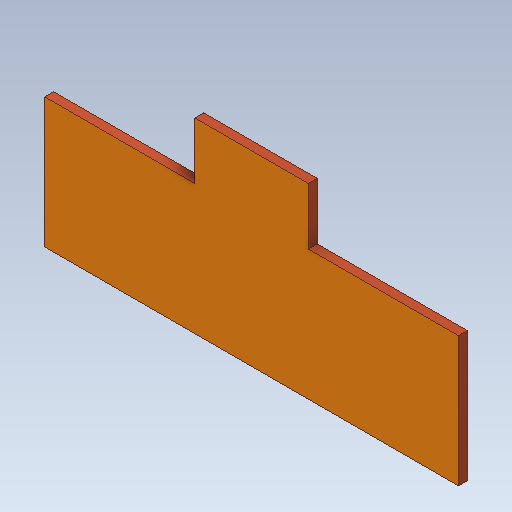
# Autodesk Inventor part: pcb sensor de cor
Saved by Autodesk Inventor 2020 (Build 240168000, 168)
## iProperties
Created: 2020-04-22
Part Number: pcb sensor de cor
Material: Genérico
Document SubType Name: Modeling
Designer: gi-se
Density: 1 g/cm^3
Appearance: Cobre - Acetinado
Author: gi-se
Autodesk Inventor part; units mm, degrees
ref_plane "YZ Plane" through (0, 0, 0) normal (1, 0, 0) x (0, 1, 0)
ref_plane "XZ Plane" through (0, 0, 0) normal (0, 1, 0) x (-1, 0, 0)
ref_plane "XY Plane" through (0, 0, 0) normal (0, 0, 1) x (1, 0, 0)
sketch "Esboço1" plane through (0, 0, 0) normal (0, 0, 1) x (1, 0, 0)
  line L0 (1.0701, 11.9834) -> (-0.8299, 11.9834)
  line L1 (-64.2299, 11.9834) -> (-64.2299, -10.0166)
  line L2 (-64.2299, -10.0166) -> (5.7701, -10.0166)
  line L3 (5.7701, -10.0166) -> (5.7701, 11.9834)
  line L4 (-61.2299, -10.5466) -> (-61.2299, 13.5834)
  line L5 (2.7701, 57.5834) -> (2.7701, -6.4166)
  line L6 (-31.3299, 21.5834) -> (-37.5299, 21.5834)
  line L7 (5.7701, -10.0166) -> (2.8701, -10.0166)
  line L8 (-59.5299, 11.9834) -> (-57.6299, 11.9834)
  line L9 (-38.8299, 21.5834) -> (-38.8299, 12.0834)
  line L10 (-19.6299, 21.5834) -> (-19.6299, 12.0834)
  line L11 (-19.6299, 11.9834) -> (-19.6299, 21.5834)
  line L12 (-19.6299, 21.5834) -> (-38.8299, 21.5834)
  line L13 (-38.8299, 21.5834) -> (-38.8299, 11.9834)
  line L14 (-64.2299, 11.9834) -> (-38.8299, 11.9834)
  line L15 (-19.6299, 11.9834) -> (5.7701, 11.9834)
  point P0 (0, 0)
extrude "Extrusão1" add sketch "Esboço1" along normal blind 1.5
